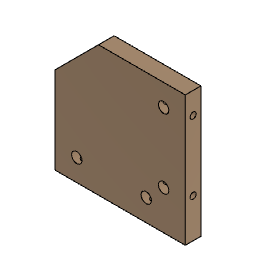
Base Brace R (Autodesk Fusion 360 design; units mm, degrees)
Autodesk Fusion 360 part; units mm, degrees
sketch "Front" plane through (0, 0, 0) normal (0, 1, 0) x (1, 0, 0)
  line L0 (0, 0) -> (-150, 0)
  line L1 (-150, 0) -> (-150, -100)
  line L2 (-100, -150) -> (0, -150)
  line L3 (0, -150) -> (0, 0)
  line L4 (-100, -150) -> (-150, -100)
  line L5 (-25, 0) -> (-25, -150) construction
  line L6 (0, -25) -> (-150, -25) construction
  circle A0 centre (-45, -25) radius 6
  circle A1 centre (-125, -25) radius 6
  circle A2 centre (-25, -45) radius 6
  circle A3 centre (-25, -125) radius 6
  dimension "d1" = 150
  dimension "d2" = 150
  dimension "d3" = 50
  dimension "d4" = 50
  dimension "d5" = 25
  dimension "d6" = 25
  dimension "d7" = 12
  dimension "d8" = 12
  dimension "d9" = 12
  dimension "d10" = 12
  dimension "d11" = 45
  dimension "d12" = 80
  dimension "d13" = 45
  dimension "d14" = 80
  constraint horizontal L0
  constraint vertical L1
  constraint horizontal L2
  constraint vertical L3
  constraint coincident L0.start L3.end
  constraint coincident L2 L5.end
  constraint perpendicular L2 L5
  constraint coincident L3 L6.start
  constraint coincident L1 L6.end
  constraint perpendicular L1 L6
  constraint coincident L6 A0.centre
  constraint coincident L6 A1.centre
  constraint coincident L5 A2.centre
  constraint coincident L5 A3.centre
  measures "d1" distance of L0.start L0.end
  measures "d2" distance of L0.start L2.end
  measures "d3" horizontal distance of L2.start L1.end
  measures "d4" vertical distance of L2.start L1.end
  measures "d5" distance of L0 L6
  measures "d6" distance of L3 L5
  measures "d7" diameter of A0
  measures "d8" diameter of A1
  measures "d9" diameter of A2
  measures "d10" diameter of A3
  measures "d11" distance of L0 A2.centre
  measures "d12" distance of A2.centre A3.centre
  measures "d13" distance of L3 A0.centre
  measures "d14" distance of A0.centre A1.centre
extrude "Extrude1" add sketch "Front" along normal blind 18
sketch "Right" plane through (0, 0, 0) normal (1, 0, 0) x (0, 1, 0)
  line L0 (0, 150) -> (0, 0)
  line L1 (0, 0) -> (18, 0)
  line L2 (18, 0) -> (18, 150)
  line L3 (18, 150) -> (0, 150)
  line L4 (9, 0) -> (9, 150) construction
  circle A0 centre (9, 45) radius 3.5
  circle A1 centre (9, 125) radius 3.5
  dimension "d17" = 7
  dimension "d18" = 7
  dimension "d19" = 45
  dimension "d20" = 80
  constraint midpoint L1 L4.start
  constraint midpoint L3 L4.end
  constraint coincident L4 A0.centre
  constraint coincident L4 A1.centre
  measures "d17" diameter of A0
  measures "d18" diameter of A1
  measures "d19" distance of L1 A0.centre
  measures "d20" distance of A0.centre A1.centre
extrude "Extrude2" cut sketch "Right" against normal blind 35 contours A0 | A1
sketch "Sketch3" plane through (0, 0, 0) normal (0, 0, -1) x (1, 0, 0)
  line L0 (0, 0) -> (-150, 0)
  line L1 (-150, 0) -> (-150, -18)
  line L2 (-150, -18) -> (0, -18)
  line L3 (0, -18) -> (0, 0)
  line L4 (0, -9) -> (-150, -9) construction
  circle A0 centre (-45, -9) radius 3.5
  circle A1 centre (-125, -9) radius 3.5
  dimension "d23" = 7
  dimension "d24" = 7
  dimension "d25" = 45
  dimension "d26" = 80
  constraint midpoint L3 L4.start
  constraint midpoint L1 L4.end
  constraint coincident L4 A0.centre
  constraint coincident L4 A1.centre
  measures "d23" diameter of A0
  measures "d24" diameter of A1
  measures "d25" distance of L3 A0.centre
  measures "d26" distance of A0.centre A1.centre
extrude "Extrude3" cut sketch "Sketch3" against normal blind 35 contours A0 | A1
named bodies: "Base Brace R"
